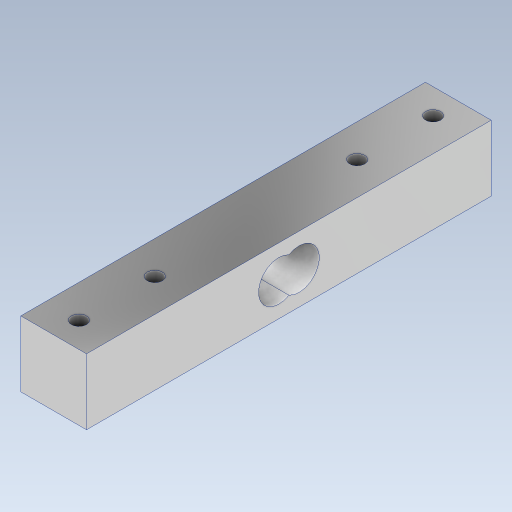
# Autodesk Inventor part: celda
Saved by Autodesk Inventor 2023 (Build 270158000, 158)
## iProperties
Created: 2023-03-18
Part Number: celda
Material: Aluminum 6061
Document SubType Name: Modeling
Designer: santi
Density: 2.7 g/cm^3
Appearance: Aluminum - Flat
Author: santi
Autodesk Inventor part; units mm, degrees
ref_plane "YZ Plane" through (0, 0, 0) normal (1, 0, 0) x (0, 1, 0)
ref_plane "XZ Plane" through (0, 0, 0) normal (0, 1, 0) x (-1, 0, 0)
ref_plane "XY Plane" through (0, 0, 0) normal (0, 0, 1) x (1, 0, 0)
sketch "Sketch1" plane through (0, 0, 0) normal (0, 1, 0) x (-1, 0, 0)
  line L0 (0, 0) -> (13, 0)
  line L1 (13, 0) -> (13, -80)
  line L2 (13, -80) -> (0, -80)
  line L3 (0, -80) -> (0, 0)
  circle A0 centre (6.5, -60) radius 1.5
  circle A1 centre (6.5, -75) radius 1.5
  circle A2 centre (6.5, -20) radius 1.5
  circle A3 centre (6.5, -5) radius 1.5
  point P0 (6.5, -80)
  point P1 (6.5, 0)
  dimension "d0" = 13
  dimension "d1" = 80
  dimension "d2" = 3
  dimension "d3" = 20
  dimension "d4" = 3
  dimension "d5" = 5
  dimension "d6" = 3
  dimension "d7" = 3
  dimension "d8" = 5
  dimension "d9" = 20
  constraints: 8 end point, 4 centre point, 4 vertical alignment, 2 midpoint, 2 parallel, 1 horizontal, 1 perpendicular
  measures "d0" distance of L1.end L2.end
  measures "d1" distance of L0.end L1.end
  measures "d2" diameter of A0
  measures "d3" vertical distance of L2.end A0.centre
  measures "d4" diameter of A1
  measures "d5" distance of point (6.5, -80) A1.centre
  measures "d6" diameter of A2
  measures "d7" diameter of A3
  measures "d8" distance from line of A3.centre L0
  measures "d9" distance from line of A2.centre L0
extrude "Extrusion1" add sketch "Sketch1" along normal blind 13
sketch "Sketch2" plane through (0, 0, 0) normal (1, 0, 0) x (0, 0, -1)
  arc A0 (40, 9.9641) -> (40, 3.0359) centre (38, 6.5) ccw
  arc A1 (40, 3.0359) -> (40, 9.9641) centre (42, 6.5) ccw
  line L0 (0, 13) -> (80, 13) construction
  line L1 (80, 0) -> (80, 13) construction
  point P0 (0, 0)
  point P1 (40, 13)
  point P2 (80, 6.5)
  point P3 (80, 6.5)
  dimension "d12" = 8
  dimension "d13" = 8
  constraints: 5 point on circle, 3 midpoint, 2 centre point, 2 horizontal alignment, 1 vertical alignment
  measures "d12" diameter of A0
  measures "d13" diameter of A1
extrude "Extrusion2" cut sketch "Sketch2" against normal blind 13
body "Solid1"
